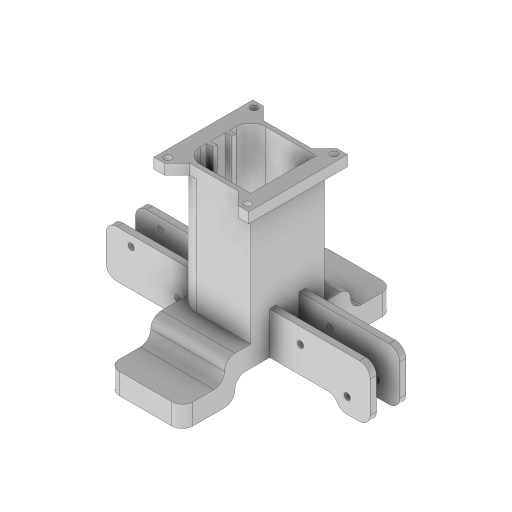
# Autodesk Inventor part: CARCASA_NUEVA
Saved by Autodesk Inventor 2024 (Build 280153000, 153)
## iProperties
Created: 2024-08-20
Part Number: CARCASA_NUEVA
Material: Generic
Document SubType Name: Modeling
Designer: Jhuliams
Density: 1 g/cm^3
Appearance: Default
Author: Jhuliams
Autodesk Inventor part; units mm, degrees
ref_plane "YZ Plane" through (0, 0, 0) normal (1, 0, 0) x (0, 1, 0)
ref_plane "XZ Plane" through (0, 0, 0) normal (0, 1, 0) x (-1, 0, 0)
ref_plane "XY Plane" through (0, 0, 0) normal (0, 0, 1) x (1, 0, 0)
sketch "Sketch1" plane through (0, 0, 0) normal (0, 1, 0) x (-1, 0, 0)
  line L0 (22.5, 50.25) -> (-22.5, 50.25)
  line L1 (-22.5, 50.25) -> (-22.5, -50.25)
  line L2 (-22.5, -50.25) -> (22.5, -50.25)
  line L3 (22.5, -50.25) -> (22.5, 50.25)
  line L4 (22.5, 50.25) -> (-22.5, -50.25) construction
  line L5 (-22.5, 50.25) -> (22.5, -50.25) construction
  line L6 (15.5, 15.5) -> (-15.5, 15.5)
  line L7 (-15.5, 15.5) -> (-15.5, -15.5)
  line L8 (-15.5, -15.5) -> (15.5, -15.5)
  line L9 (15.5, -15.5) -> (15.5, 15.5)
  line L10 (15.5, 15.5) -> (-15.5, -15.5) construction
  line L11 (-15.5, 15.5) -> (15.5, -15.5) construction
  line L12 (0, 15.5) -> (11.5, 15.5)
  line L13 (22.5, 50.25) -> (17.5, 50.25)
  line L14 (0, 0) -> (7.9375, 0)
  line L15 (-22.5, -50.25) -> (-22.5, -47.25)
  point P0 (11.5, -15.5)
  point P1 (-11.5, -15.5)
  point P2 (0, -15.5)
  dimension "d0" = 45
  dimension "d1" = 100.5
  dimension "d2" = 31
  dimension "d3" = 31
  constraints: 32 end point, 6 midpoint, 4 parallel, 3 horizontal, 3 point on line, 2 perpendicular, 1 symmetric about line
  measures "d0" distance of L2.end L1.end
  measures "d1" distance of L1.end L0.end
  measures "d2" distance of L8.end L7.end
  measures "d3" distance of L7.end L6.end
extrude "Extrusion1" add sketch "Sketch1" along normal blind 5
fillet "Fillet1" radius 7 2 edges at (-15.5, 2.5, 15.5) (15.5, 2.5, 15.5)
sketch "Sketch2" plane through (0, 0, 0) normal (0, -1, 0) x (1, 0, 0)
  line L0 (17.5, 17.5) -> (-17.5, 17.5)
  line L1 (-17.5, 17.5) -> (-17.5, -17.5)
  line L2 (-17.5, -17.5) -> (17.5, -17.5)
  line L3 (17.5, -17.5) -> (17.5, 17.5)
  line L4 (17.5, 17.5) -> (-17.5, -17.5) construction
  line L5 (-17.5, 17.5) -> (17.5, -17.5) construction
  line L6 (22.5, -50.25) -> (-22.5, -50.25) projected
  line L7 (22.5, 50.25) -> (22.5, -50.25) projected
  line L8 (-22.5, 50.25) -> (22.5, 50.25) projected
  line L9 (-22.5, -50.25) -> (-22.5, 50.25) projected
  arc A0 (15.5, 8.5) -> (8.5, 15.5) centre (8.5, 8.5) ccw projected
  line L10 (15.5, -15.5) -> (15.5, 8.5) projected
  line L11 (-15.5, -15.5) -> (15.5, -15.5) projected
  line L12 (-15.5, 8.5) -> (-15.5, -15.5) projected
  arc A1 (-8.5, 15.5) -> (-15.5, 8.5) centre (-8.5, 8.5) ccw projected
  line L13 (8.5, 15.5) -> (-8.5, 15.5) projected
  point P0 (0, 0)
  dimension "d24" = 35
  dimension "d25" = 35
  constraints: 12 end point, 2 midpoint, 2 parallel, 1 horizontal, 1 perpendicular
  measures "d24" distance of L2.end L1.end
  measures "d25" distance of L1.end L0.end
extrude "Extrusion2" add sketch "Sketch2" along normal blind 65 contours L3 L2 L1 L0
sketch "Sketch3" plane through (0, 5, 0) normal (0, 1, 0) x (1, 0, 0)
  line L0 (0, 0) -> (0, -15.5)
  line L1 (8.5, -15.5) -> (-8.5, -15.5) projected
  line L2 (0, -15.5) -> (-3.5, -15.5)
  line L3 (-3.5, -15.5) -> (-5.5, -15.5)
  line L4 (-5.5, -15.5) -> (-5.5, -12.5)
  line L5 (-5.5, -12.5) -> (-3.5, -12.5)
  line L6 (-3.5, -12.5) -> (-3.5, -15.5)
  line L7 (3.5, -15.5) -> (5.5, -15.5)
  line L8 (5.5, -15.5) -> (5.5, -12.5)
  line L9 (5.5, -12.5) -> (3.5, -12.5)
  line L10 (3.5, -12.5) -> (3.5, -15.5)
  dimension "d28" = 3.5
  dimension "d29" = 2
  dimension "d30" = 3
  constraints: 20 end point, 4 symmetric about line, 2 parallel, 1 horizontal, 1 midpoint, 1 perpendicular, 1 point on line
  measures "d28" distance of L0.end L2.end
  measures "d29" distance of L4.end L5.end
  measures "d30" distance of L3.end L4.end
extrude "Extrusion3" add sketch "Sketch3" against normal blind 70
fillet "Fillet2" radius 9 2 edges at (-17.5, -32.5, 17.5) (17.5, -32.5, 17.5)
sketch "Sketch8" plane through (0, 5, 0) normal (0, 1, 0) x (1, 0, 0)
  line L0 (-15.5, -15.5) -> (15.5, -15.5)
  line L1 (15.5, -15.5) -> (15.5, 15.5)
  line L2 (15.5, 15.5) -> (-15.5, 15.5)
  line L3 (-15.5, 15.5) -> (-15.5, -15.5)
  line L4 (-15.5, -15.5) -> (15.5, 15.5) construction
  line L5 (15.5, -15.5) -> (-15.5, 15.5) construction
  point P0 (0, 0)
  dimension "d45" = 31
  dimension "d46" = 31
  constraints: 12 end point, 2 midpoint, 2 parallel, 1 horizontal, 1 perpendicular
  measures "d45" distance of L2.end L1.end
  measures "d46" distance of L1.end L0.end
extrude "Extrusion8" cut sketch "Sketch8" against normal blind 5
sketch "Sketch9" plane through (0, 5, 0) normal (0, 1, 0) x (1, 0, 0)
  line L0 (15.5, -15.5) -> (-15.5, -15.5) projected
  line L1 (-15.5, -15.5) -> (-15.5, 15.5) projected
  line L2 (-15.5, 15.5) -> (15.5, 15.5) projected
  line L3 (15.5, 15.5) -> (15.5, -15.5) projected
  circle A0 centre (0, 0) radius 13
  dimension "d49" = 26
  constraints: 1 centre point, 1 coincident
  measures "d49" diameter of A0
extrude "Extrusion9" add sketch "Sketch9" against normal blind 5
sketch "Sketch11" plane through (0, -65, 0) normal (0, -1, 0) x (1, 0, 0)
  line L0 (-23.5, 22.5) -> (23.5, 22.5)
  line L1 (23.5, 22.5) -> (23.5, -22.5)
  line L2 (23.5, -22.5) -> (-23.5, -22.5)
  line L3 (-23.5, -22.5) -> (-23.5, 22.5)
  line L4 (-23.5, 22.5) -> (23.5, -22.5) construction
  line L5 (23.5, 22.5) -> (-23.5, -22.5) construction
  arc A0 (17.5, 8.5) -> (8.5, 17.5) centre (8.5, 8.5) ccw projected
  line L6 (8.5, 17.5) -> (-8.5, 17.5) projected
  arc A1 (-8.5, 17.5) -> (-17.5, 8.5) centre (-8.5, 8.5) ccw projected
  line L7 (-17.5, 8.5) -> (-17.5, -17.5) projected
  line L8 (-17.5, -17.5) -> (17.5, -17.5) projected
  line L9 (17.5, -17.5) -> (17.5, 8.5) projected
  line L10 (15.5, 8.5) -> (15.5, -15.5) projected
  line L11 (15.5, -15.5) -> (-15.5, -15.5) projected
  line L12 (-15.5, -15.5) -> (-15.5, 8.5) projected
  arc A2 (-8.5, 15.5) -> (-15.5, 8.5) centre (-8.5, 8.5) ccw projected
  line L13 (-8.5, 15.5) -> (-5.5, 15.5) projected
  line L14 (-3.5, 15.5) -> (3.5, 15.5) projected
  line L15 (5.5, 15.5) -> (8.5, 15.5) projected
  arc A3 (15.5, 8.5) -> (8.5, 15.5) centre (8.5, 8.5) ccw projected
  line L16 (-23.5, 22.5) -> (-23.5, 17.5)
  line L17 (0, 0) -> (-17.5, 0)
  line L18 (-17.5, 0) -> (-17.5, 11.5)
  line L19 (-17.5, 11.5) -> (-23.5, 17.5)
  line L20 (0, 0) -> (0, 8.5)
  line L21 (17.5, 11.5) -> (23.5, 17.5)
  line L22 (-17.5, -11.5) -> (-23.5, -17.5)
  line L23 (17.5, -11.5) -> (23.5, -17.5)
  line L24 (0, 0) -> (17.5, 0)
  line L25 (17.5, 11.5) -> (17.5, 0)
  line L26 (-5.5, 15.5) -> (-5.5, 12.5) projected
  line L27 (-5.5, 12.5) -> (-3.5, 12.5) projected
  line L28 (-3.5, 12.5) -> (-3.5, 15.5) projected
  line L29 (3.5, 15.5) -> (3.5, 12.5) projected
  line L30 (3.5, 12.5) -> (5.5, 12.5) projected
  line L31 (5.5, 12.5) -> (5.5, 15.5) projected
  dimension "d61" = 47
  dimension "d62" = 45
  dimension "d63" = 5
  dimension "d65" = 11.5
  constraints: 32 end point, 6 symmetric about line, 4 perpendicular, 4 point on line, 2 midpoint, 2 parallel, 1 horizontal, 1 vertical
  measures "d61" distance of L1.end L2.end
  measures "d62" distance of L0.end L1.end
  measures "d63" distance of L0.start L16.end
  measures "d65" distance of L17.end L18.end
extrude "Extrusion11" add sketch "Sketch11" against normal blind 5 contours L0 L1 L21 L25 A0 L6 A1 L18 L19 L3 | L22 L7 L8 L9 L23 L1 L2 L3
sketch "Sketch12" plane through (0, -65, 0) normal (0, -1, 0) x (1, 0, 0)
  line L0 (23.5, 22.5) -> (20.5, 22.5)
  line L1 (-23.5, 22.5) -> (23.5, 22.5) projected
  line L2 (20.5, 22.5) -> (20.5, 19)
  circle A0 centre (20.5, 19) radius 1.65
  line L3 (-20.5, -19) -> (20.5, -19)
  line L4 (20.5, -19) -> (20.5, 19)
  line L5 (20.5, 19) -> (-20.5, 19)
  line L6 (-20.5, 19) -> (-20.5, -19)
  line L7 (-20.5, -19) -> (20.5, 19) construction
  line L8 (20.5, -19) -> (-20.5, 19) construction
  circle A1 centre (-20.5, 19) radius 1.65
  circle A2 centre (20.5, -19) radius 1.65
  circle A3 centre (-20.5, -19) radius 1.65
  point P0 (0, 0)
  dimension "d68" = 3
  dimension "d69" = 3.5
  dimension "d70" = 90
  dimension "d71" = 3.3
  dimension "d74" = 41
  dimension "d77" = 38
  constraints: 16 end point, 4 centre point, 2 horizontal, 2 midpoint, 2 parallel, 2 perpendicular, 1 coincident, 1 point on line, 1 vertical, 6 other
  measures "d68" distance of L0.start L0.end
  measures "d69" distance of L0.end L2.end
  measures "d70" angle of L2 L0
  measures "d71" diameter of A0
  measures "d74" distance of L4.end A1.centre
  measures "d77" distance of L4.end A2.centre
extrude "Extrusion12" cut sketch "Sketch12" against normal blind 6 contours A0 L4 L2 | L2 L5 A0 | L4 A0 L5 | A1 L6 L5 | L5 L6 A1 | A2 L3 L4 | L4 L3 A2 | A3 L3 L6 | L6 L3 A3
sketch "Sketch15" plane through (0, 0, 0) normal (0, -1, 0) x (1, 0, 0)
  line L0 (17.5, -17.5) -> (-17.5, -17.5) projected
  line L1 (5.5, -83) -> (-5.5, -83)
  line L2 (-5.5, -83) -> (-5.5, -17.5)
  line L3 (-5.5, -17.5) -> (5.5, -17.5)
  line L4 (5.5, -17.5) -> (5.5, -83)
  line L5 (22.5, -50.25) -> (-22.5, -50.25) projected
  line L6 (5.5, -83) -> (-5.5, -17.5) construction
  line L7 (-5.5, -83) -> (5.5, -17.5) construction
  point P0 (0, 0)
  point P1 (0, -50.25)
  point P2 (-5.5, -50.25)
  point P3 (5.5, -50.25)
  dimension "d94" = 11
  constraints: 12 end point, 3 midpoint, 2 parallel, 1 horizontal, 1 perpendicular, 1 point on line
  measures "d94" distance of L2.end L3.end
extrude "Extrusion15" cut sketch "Sketch15" against normal blind 8 contours L4 L5 L2 L0
sketch "Sketch16" plane through (0, 0, 0) normal (0, -1, 0) x (1, 0, 0)
  line L0 (5.5, -17.5) -> (5.5, -50.25) projected
  line L1 (5.5, -50.25) -> (8.5, -50.25)
  line L2 (8.5, -50.25) -> (8.5, -17.5)
  line L3 (8.5, -17.5) -> (5.5, -17.5)
  line L4 (5.5, -17.5) -> (5.5, -50.25)
  line L5 (0, 0) -> (0, -4.7625)
  line L6 (-5.5, -17.5) -> (-5.5, -50.25)
  line L7 (-5.5, -50.25) -> (-8.5, -50.25)
  line L8 (-8.5, -50.25) -> (-8.5, -17.5)
  line L9 (-8.5, -17.5) -> (-5.5, -17.5)
  line L10 (-5.5, -17.5) -> (-5.5, -50.25)
  line L11 (5.5, -50.25) -> (8.5, -50.25)
  line L12 (8.5, -50.25) -> (8.5, -65.25)
  line L13 (8.5, -65.25) -> (5.5, -65.25)
  line L14 (5.5, -65.25) -> (5.5, -50.25)
  line L15 (-8.5, -50.25) -> (-8.5, -65.25)
  line L16 (-8.5, -65.25) -> (-5.5, -65.25)
  line L17 (-5.5, -65.25) -> (-5.5, -50.25)
  dimension "d97" = 3
  dimension "d98" = 32.75
  dimension "d101" = 15
  constraints: 34 end point, 8 symmetric about line, 4 parallel, 2 horizontal, 2 perpendicular
  measures "d97" distance of L3.end L2.end
  measures "d98" distance of L2.end L1.end
  measures "d101" distance of L11.end L12.end
extrude "Extrusion16" add sketch "Sketch16" along normal blind 15
sketch "Sketch17" plane through (0, 0, 0) normal (0, 1, 0) x (1, 0, 0)
  line L0 (-5.5, 50.25) -> (-8.5, 50.25) projected
  line L1 (-5.5, 65.25) -> (-5.5, 50.25) projected
  line L2 (-8.5, 65.25) -> (-5.5, 65.25) projected
  line L3 (-8.5, 50.25) -> (-8.5, 65.25) projected
  line L4 (8.5, 50.25) -> (5.5, 50.25) projected
  line L5 (8.5, 65.25) -> (8.5, 50.25) projected
  line L6 (5.5, 65.25) -> (8.5, 65.25) projected
  line L7 (5.5, 50.25) -> (5.5, 65.25) projected
  point P0 (0, 0)
extrude "Extrusion17" add sketch "Sketch17" along normal blind 10
sketch "Sketch18" plane through (-8.5, 0, -50.25) normal (-1, 0, 0) x (0, 0, 1)
  circle A0 centre (-4.1, 2.65) radius 1.5 projected
  circle A1 centre (18.1, -7.65) radius 1.5 projected
  point P0 (50.25, 0)
extrude "Extrusion18" cut sketch "Sketch18" against normal blind 20
mirror "Mirror1" about plane through (0, 0, 0) normal (0, 0, 1) of "Extrusion15"
sketch "Sketch20" plane through (-8.5, -60, 17.5) normal (0, 0, 1) x (1, 0, 0)
  line L0 (-4.5, 65) -> (21.5, 65) projected
  line L1 (8.5, 65) -> (8.5, 50)
  line L2 (5, -5) -> (5, 60) projected
  line L3 (12, 40) -> (5, 40)
  line L4 (5, 40) -> (5, 60)
  line L5 (5, 60) -> (12, 60)
  line L6 (12, 60) -> (12, 40)
  line L7 (12, 40) -> (5, 60) construction
  line L8 (5, 40) -> (12, 60) construction
  line L9 (8.5, 60) -> (8.5, 52)
  line L10 (8.5, 52) -> (5, 52)
  line L11 (8.5, 52) -> (12, 52)
  dimension "d106" = 15
  dimension "d107" = 7
  dimension "d108" = 20
  dimension "d129" = 8
  constraints: 20 end point, 3 midpoint, 3 perpendicular, 3 point on line, 2 parallel, 1 horizontal, 1 vertical
  measures "d106" distance of L1.start L1.end
  measures "d107" distance of L2.end L5.end
  measures "d108" distance of L3.end L2.end
  measures "d129" distance of L9.start L9.end
extrude "Extrusion19" cut sketch "Sketch20" against normal blind 7 contours L11 L6 L3 L2 L10
sketch "Sketch21" plane through (0, 0, 0) normal (0, -1, 0) x (1, 0, 0)
  line L0 (5.5, 50.25) -> (5.5, 17.5) projected
  line L1 (5.5, 50.25) -> (8.5, 50.25)
  line L2 (8.5, 50.25) -> (8.5, 17.5)
  line L3 (8.5, 17.5) -> (5.5, 17.5)
  line L4 (5.5, 17.5) -> (5.5, 50.25)
  line L5 (0, 0) -> (0, 5.2577)
  line L6 (-5.5, 50.25) -> (-5.5, 17.5)
  line L7 (-5.5, 50.25) -> (-8.5, 50.25)
  line L8 (-8.5, 50.25) -> (-8.5, 17.5)
  line L9 (-8.5, 17.5) -> (-5.5, 17.5)
  line L10 (-5.5, 17.5) -> (-5.5, 50.25)
  line L11 (5.5, 50.25) -> (8.5, 50.25)
  line L12 (8.5, 50.25) -> (8.5, 60.25)
  line L13 (8.5, 60.25) -> (5.5, 60.25)
  line L14 (5.5, 60.25) -> (5.5, 50.25)
  line L15 (-8.5, 50.25) -> (-8.5, 60.25)
  line L16 (-8.5, 60.25) -> (-5.5, 60.25)
  line L17 (-5.5, 60.25) -> (-5.5, 50.25)
  dimension "d111" = 3
  dimension "d112" = 32.75
  dimension "d120" = 3
  dimension "d121" = 10
  constraints: 34 end point, 8 symmetric about line, 4 parallel, 2 horizontal, 2 perpendicular, 1 vertical
  measures "d111" distance of L2.end L3.end
  measures "d112" distance of L1.end L2.end
  measures "d120" distance of L13.end L12.end
  measures "d121" distance of L12.end L11.end
extrude "Extrusion20" add sketch "Sketch21" along normal mid plane 25
sketch "Sketch23" plane through (0, 5, 0) normal (0, 1, 0) x (1, 0, 0)
  line L0 (-12.5, 25.5) -> (12.5, 25.5)
  line L1 (12.5, 25.5) -> (12.5, -25.5)
  line L2 (12.5, -25.5) -> (-12.5, -25.5)
  line L3 (-12.5, -25.5) -> (-12.5, 25.5)
  line L4 (-12.5, 25.5) -> (12.5, -25.5) construction
  line L5 (12.5, 25.5) -> (-12.5, -25.5) construction
  point P0 (0, 0)
  dimension "d115" = 25
  dimension "d116" = 51
  constraints: 12 end point, 2 midpoint, 2 parallel, 1 horizontal, 1 perpendicular
  measures "d115" distance of L1.end L2.end
  measures "d116" distance of L0.end L1.end
extrude "Extrusion21" cut sketch "Sketch23" along normal blind 10
sketch "Sketch24" plane through (8.5, 0, 50.25) normal (1, 0, 0) x (0, 0, -1)
  circle A0 centre (1.9, -7.65) radius 1.5 projected
  circle A1 centre (24.1, 2.65) radius 1.5 projected
  point P0 (50.25, 0)
extrude "Extrusion22" cut sketch "Sketch24" against normal blind 25
sketch "Sketch25" plane through (0, 0, 0) normal (0, -1, 0) x (1, 0, 0)
  line L0 (8.5, 50.25) -> (8.5, 17.5) projected
  arc A0 (17.5, 8.5) -> (8.5, 17.5) centre (8.5, 8.5) ccw projected
  line L1 (17.5, 8.5) -> (17.5, -17.5) projected
  line L2 (17.5, -17.5) -> (8.5, -17.5) projected
  line L3 (8.5, -17.5) -> (8.5, -50.25) projected
  line L4 (22.5, -50.25) -> (8.5, -50.25) projected
  line L5 (22.5, 50.25) -> (22.5, -50.25) projected
  line L6 (8.5, 50.25) -> (22.5, 50.25) projected
  line L7 (-8.5, 17.5) -> (-8.5, 50.25) projected
  line L8 (-22.5, 50.25) -> (-8.5, 50.25) projected
  line L9 (-22.5, -50.25) -> (-22.5, 50.25) projected
  line L10 (-8.5, -50.25) -> (-22.5, -50.25) projected
  line L11 (-8.5, -50.25) -> (-8.5, -17.5) projected
  line L12 (-8.5, -17.5) -> (-17.5, -17.5) projected
  line L13 (-17.5, -17.5) -> (-17.5, 8.5) projected
  arc A1 (-8.5, 17.5) -> (-17.5, 8.5) centre (-8.5, 8.5) ccw projected
  point P0 (0, 0)
extrude "Extrusion23" cut sketch "Sketch25" against normal blind 25
sketch "Sketch26" plane through (0, 12.5, 0) normal (0, 1, 0) x (1, 0, 0)
  line L0 (-5.5, -25.5) -> (-8.5, -25.5) projected
  line L1 (-8.5, -25.5) -> (-8.5, -60.25) projected
  line L2 (-8.5, -60.25) -> (-5.5, -60.25) projected
  line L3 (-5.5, -60.25) -> (-5.5, -25.5) projected
  line L4 (8.5, -25.5) -> (5.5, -25.5) projected
  line L5 (5.5, -25.5) -> (5.5, -60.25) projected
  line L6 (5.5, -60.25) -> (8.5, -60.25) projected
  line L7 (8.5, -60.25) -> (8.5, -25.5) projected
  point P0 (0, 0)
extrude "Extrusion24" cut sketch "Sketch26" against normal blind 2.5
fillet "Fillet4" radius 5 16 edges at (-7, 5, 25.5) (-7, 10, 25.5) (7, 5, 25.5) (7, 10, 25.5) (-7, 5, -50.25) (-7, 10, -50.25) (7, 10, -50.25) (7, 5, -50.25) (7, 10, -65.25) (-7, 10, -65.25) (-7, -15, -65.25) (7, -15, -65.25) (-7, 10, 60.25) (7, 10, 60.25) (7, -12.5, 60.25) (-7, -12.5, 60.25)
sketch "Sketch27" plane through (0, 5, 0) normal (0, 1, 0) x (1, 0, 0)
  line L0 (-50, -17.5) -> (50, -17.5)
  line L1 (50, -17.5) -> (50, 17.5)
  line L2 (50, 17.5) -> (-50, 17.5)
  line L3 (-50, 17.5) -> (-50, -17.5)
  line L4 (-50, -17.5) -> (50, 17.5) construction
  line L5 (50, -17.5) -> (-50, 17.5) construction
  circle A0 centre (0, 0) radius 13 projected
  line L6 (5.5, 45.25) -> (8.5, 45.25) projected
  line L7 (5.5, 45.25) -> (5.5, 17.5) projected
  line L8 (5.5, 17.5) -> (-5.5, 17.5) projected
  line L9 (-5.5, 17.5) -> (-5.5, 45.25) projected
  line L10 (-8.5, 45.25) -> (-5.5, 45.25) projected
  line L11 (-8.5, 45.25) -> (-8.5, 17.5) projected
  line L12 (-8.5, 17.5) -> (-17.5, 17.5) projected
  line L13 (-17.5, 17.5) -> (-17.5, -8.5) projected
  arc A1 (-17.5, -8.5) -> (-8.5, -17.5) centre (-8.5, -8.5) ccw projected
  line L14 (-8.5, -17.5) -> (-8.5, -20.5) projected
  line L15 (-5.5, -20.5) -> (-8.5, -20.5) projected
  line L16 (-5.5, -17.5) -> (-5.5, -20.5) projected
  line L17 (-5.5, -17.5) -> (5.5, -17.5) projected
  line L18 (5.5, -20.5) -> (5.5, -17.5) projected
  line L19 (8.5, -20.5) -> (5.5, -20.5) projected
  line L20 (8.5, -20.5) -> (8.5, -17.5) projected
  arc A2 (8.5, -17.5) -> (17.5, -8.5) centre (8.5, -8.5) ccw projected
  line L21 (17.5, -8.5) -> (17.5, 17.5) projected
  line L22 (17.5, 17.5) -> (8.5, 17.5) projected
  line L23 (8.5, 17.5) -> (8.5, 45.25) projected
  dimension "d130" = 100
  constraints: 12 end point, 2 midpoint, 2 parallel, 1 horizontal, 1 perpendicular
  measures "d130" distance of L2.end L1.end
extrude "Extrusion25" add sketch "Sketch27" along normal mid plane 20 contours L3 L2 L13 A1 L0 | A2 L21 L2 L1 L0
sketch "Sketch28" plane through (0, 15, 0) normal (0, 1, 0) x (1, 0, 0)
  line L0 (-25, 20) -> (25, 20)
  line L1 (25, 20) -> (25, -20)
  line L2 (25, -20) -> (-25, -20)
  line L3 (-25, -20) -> (-25, 20)
  line L4 (-25, 20) -> (25, -20) construction
  line L5 (25, 20) -> (-25, -20) construction
  point P0 (0, 0)
  dimension "d133" = 50
  dimension "d134" = 40
  constraints: 12 end point, 2 midpoint, 2 parallel, 1 horizontal, 1 perpendicular
  measures "d133" distance of L1.end L2.end
  measures "d134" distance of L0.end L1.end
extrude "Extrusion26" cut sketch "Sketch28" against normal blind 10
sketch "Sketch29" plane through (0, -5, 0) normal (0, -1, 0) x (1, 0, 0)
  line L0 (0, 0) -> (-50, 0)
  line L1 (-50, -17.5) -> (-50, 17.5) projected
  line L2 (-70, 25) -> (-30, 25)
  line L3 (-30, 25) -> (-30, -25)
  line L4 (-30, -25) -> (-70, -25)
  line L5 (-70, -25) -> (-70, 25)
  line L6 (-70, 25) -> (-30, -25) construction
  line L7 (-30, 25) -> (-70, -25) construction
  line L8 (0, 0) -> (0, 7.9375)
  line L9 (50, -17.5) -> (50, 17.5)
  line L10 (70, 25) -> (30, 25)
  line L11 (30, 25) -> (30, -25)
  line L12 (30, -25) -> (70, -25)
  line L13 (70, -25) -> (70, 25)
  line L14 (70, 25) -> (30, -25) construction
  line L15 (30, 25) -> (70, -25) construction
  point P0 (50, 0)
  dimension "d137" = 40
  dimension "d138" = 50
  constraints: 30 end point, 7 symmetric about line, 3 midpoint, 2 parallel, 1 horizontal, 1 perpendicular, 1 vertical
  measures "d137" distance of L3.end L4.end
  measures "d138" distance of L2.end L3.end
extrude "Extrusion27" cut sketch "Sketch29" against normal blind 10
fillet "Fillet5" radius 5 12 edges at (-30, -5, 0) (-30, 5, 0) (-25, 5, 0) (-25, 15, 0) (25, 5, 0) (25, 15, 0) (30, 5, 0) (30, -5, 0) (50, 10, -17.5) (50, 10, 17.5) (-50, 10, -17.5) (-50, 10, 17.5)
body "Solid1"
